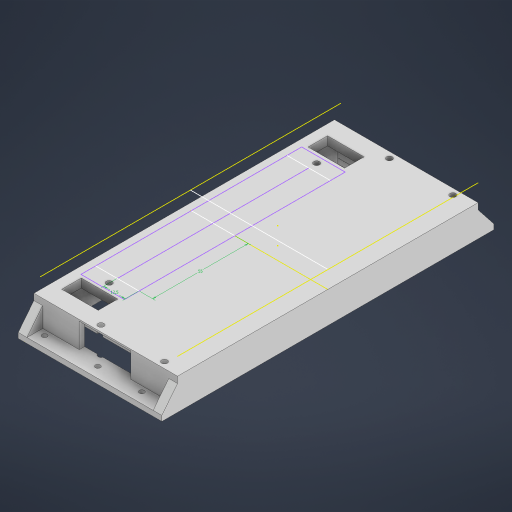
# Autodesk Inventor part: atap
Saved by Autodesk Inventor 2024.3 (Build 283343000, 343)
## iProperties
Created: 2025-06-23
Part Number: atap
Material: Generic
Document SubType Name: Modeling
Designer: Akbar Syihabuddin
Density: 1 g/cm^3
Appearance: Default
Author: Akbar Syihabuddin
Autodesk Inventor part; units mm, degrees
ref_plane "YZ Plane" through (0, 0, 0) normal (1, 0, 0) x (0, 1, 0)
ref_plane "XZ Plane" through (0, 0, 0) normal (0, 1, 0) x (-1, 0, 0)
ref_plane "XY Plane" through (0, 0, 0) normal (0, 0, 1) x (1, 0, 0)
sketch "Sketch1" plane through (0, 0, 0) normal (0, 1, 0) x (-1, 0, 0)
  line L0 (-36.0847, -75.9608) -> (-36.0847, -87.9608)
  line L1 (-36.0847, -87.9608) -> (42.9536, -87.9608)
  line L2 (42.9536, -87.9608) -> (42.9536, -75.9608)
  line L3 (42.9536, -75.9608) -> (-36.0847, -75.9608)
  line L4 (-36.0847, -75.9608) -> (-36.0847, -87.9608)
  circle A0 centre (-18.6075, -81.9608) radius 1.4
  circle A1 centre (-18.6075, -81.9608) radius 1.4
  circle A2 centre (6.6962, -81.9608) radius 1.4
  circle A3 centre (6.6962, -81.9608) radius 1.4
  circle A4 centre (37.2679, -81.9608) radius 1.4
  circle A5 centre (37.2679, -81.9608) radius 1.4
  line L5 (-36.0847, 90.7296) -> (-36.0847, 102.7296)
  line L6 (-36.0847, 102.7296) -> (42.9536, 102.7296)
  line L7 (42.9536, 102.7296) -> (42.9536, 90.7296)
  line L8 (42.9536, 90.7296) -> (-36.0847, 90.7296)
  line L9 (-36.0847, 90.7296) -> (-36.0847, 102.7296)
  circle A6 centre (-18.6075, 96.7296) radius 1.4
  circle A7 centre (-18.6075, 96.7296) radius 1.4
  circle A8 centre (6.6962, 96.7296) radius 1.4
  circle A9 centre (6.6962, 96.7296) radius 1.4
  circle A10 centre (37.2679, 96.7296) radius 1.4
  circle A11 centre (37.2679, 96.7296) radius 1.4
  point P0 (0, 0)
  point P1 (-48.8522, 7.3844)
  constraints: 20 end point, 12 centre point, 6 coincident, 2 parallel, 1 horizontal, 1 perpendicular
extrude "Extrusion1" add sketch "Sketch1" along normal blind 3
sketch "Sketch2" plane through (0, 3, 0) normal (0, 1, 0) x (1, 0, 0)
  line L0 (36.0847, -90.7296) -> (-42.9536, -90.7296) projected
  line L1 (-42.9536, -90.7296) -> (-42.9536, -102.7296) projected
  line L2 (36.0847, -90.7296) -> (-42.9536, -90.7296)
  line L3 (-42.9536, -90.7296) -> (-42.9536, -93.7296)
  line L4 (-42.9536, -93.7296) -> (36.0847, -93.7296)
  line L5 (36.0847, -93.7296) -> (36.0847, -90.7296)
  line L6 (-42.9536, 76.0091) -> (36.0847, 76.0091)
  line L7 (36.0847, 76.0091) -> (36.0847, 79.0091)
  line L8 (36.0847, 79.0091) -> (-42.9536, 79.0091)
  line L9 (-42.9536, 79.0091) -> (-42.9536, 76.0091)
  point P0 (0, 0)
  dimension "d2" = 3
  dimension "d3" = 3
  constraints: 16 end point, 4 parallel, 3 point on line, 2 horizontal, 2 perpendicular
  measures "d2" distance of L3.end L2.end
  measures "d3" distance of L7.end L6.end
extrude "Extrusion2" add sketch "Sketch2" along normal blind 25
sketch "Sketch3" plane through (-42.9536, 3, -76.0091) normal (0, 0, 1) x (1, 0, 0)
  line L0 (0, 0) -> (0, 25) projected
  line L1 (79.0383, 0) -> (79.0383, 25) projected
  line L2 (0, 25) -> (79.0383, 25)
  line L3 (79.0383, 25) -> (79.0383, 20)
  line L4 (79.0383, 20) -> (0, 20)
  line L5 (0, 20) -> (0, 25)
  point P0 (42.9536, -3)
  point P1 (0, 20)
  dimension "d6" = 5
  constraints: 8 end point, 2 parallel, 1 horizontal, 1 perpendicular, 1 point on line
  measures "d6" distance of L2.end L3.end
extrude "Extrusion3" add sketch "Sketch3" along normal blind 168
sketch "Sketch4" plane through (-42.9536, 3, 93.7296) normal (0, 0, 1) x (1, 0, 0)
  line L0 (79.0383, 0) -> (0, 0) projected
  line L1 (22.5307, 0) -> (52.1586, 0)
  line L2 (52.1586, 0) -> (52.1586, 14.1048)
  line L3 (52.1586, 14.1048) -> (22.5307, 14.1048)
  line L4 (22.5307, 14.1048) -> (22.5307, 0)
  point P0 (42.9536, -3)
  constraints: 8 end point, 2 parallel, 1 horizontal, 1 perpendicular, 1 point on line
extrude "Extrusion4" cut sketch "Sketch4" against normal blind 20
sketch "Sketch5" plane through (36.0847, 0, 102.7296) normal (1, 0, 0) x (0, 0, -1)
  line L0 (0, 3) -> (9, 3) projected
  line L1 (0, 3) -> (9, 14.3829)
  line L2 (9, 3) -> (9, 28) projected
  line L3 (0, 0) -> (0, 3) projected
  line L4 (0, 3) -> (9, 3)
  line L5 (9, 14.3829) -> (9, 3)
  point P0 (102.7296, 0)
  constraints: 6 end point, 2 collinear, 1 point on line
extrude "Extrusion5" add sketch "Sketch5" against normal blind 5
sketch "Sketch7" plane through (36.0847, 0, 102.7296) normal (1, 0, 0) x (0, 0, -1)
  line L0 (190.7387, 3) -> (181.7387, 14.3829)
  line L1 (181.7387, 14.3829) -> (190.7387, 3)
  line L2 (181.7387, 3) -> (190.7387, 3)
  line L3 (190.7387, 3) -> (181.7387, 3)
  line L4 (181.7387, 3) -> (181.7387, 14.3829)
  point P0 (102.7296, 0)
  constraints: 10 end point, 1 collinear, 1 horizontal, 1 perpendicular
extrude "Extrusion7" add sketch "Sketch7" against normal blind 5
sketch "Sketch10" plane through (36.0847, 3, -76.0091) normal (0, 0, 1) x (1, 0, 0)
  line L0 (0, -3) -> (0, 0) projected
  line L1 (0, 20) -> (-79.0383, 20) projected
  line L2 (0, -3) -> (-5, -3)
  line L3 (-5, -3) -> (-5, 20)
  line L4 (-5, 20) -> (0, 20)
  line L5 (0, 20) -> (0, -3)
  point P0 (-36.0847, -3)
  point P1 (-74.0383, 20)
  dimension "d22" = 5
  constraints: 8 end point, 2 parallel, 1 horizontal, 1 perpendicular, 1 point on line
  measures "d22" distance of L3.end L4.end
extrude "Extrusion10" add sketch "Sketch10" along normal blind 168
sketch "Sketch11" plane through (0, 28, 0) normal (0, 1, 0) x (1, 0, 0)
  line L0 (-42.9536, 79.0091) -> (-42.9536, -93.7296) projected
  line L1 (-42.9536, -7.3603) -> (36.0847, -7.3603)
  line L2 (36.0847, -93.7296) -> (36.0847, 79.0091) projected
  point P0 (0, 0)
  constraints: 2 end point, 2 midpoint
sketch "Sketch12" plane through (-42.9536, 0, -87.9608) normal (-1, 0, 0) x (0, 0, 1)
  line L0 (0, 0) -> (190.6905, 0) projected
  line L1 (0, 0) -> (0, 3) projected
  line L2 (0, 0) -> (0, 3)
  point P0 (87.9608, 0)
  constraints: 2 end point, 1 vertical
sketch "Sketch13" plane through (-42.9536, 0, 90.7296) normal (-1, 0, 0) x (0, 0, 1)
  line L0 (-178.6905, 0) -> (-178.6905, 3) projected
  line L1 (-178.6905, 0) -> (-178.6905, 3)
  line L2 (-169.7387, 3) -> (-169.7387, 28) projected
  line L3 (-178.6905, 3) -> (-169.7387, 3)
  line L4 (-169.7387, 28) -> (3, 28) projected
  line L5 (-169.7387, 3) -> (-169.7387, 28)
  line L6 (-169.7387, 28) -> (3, 28)
  line L7 (3, 28) -> (3, 3)
  line L8 (12, 0) -> (12, 3) projected
  line L9 (3, 3) -> (12, 3)
  line L10 (12, 3) -> (12, 0)
  line L11 (0, 23) -> (0, 0) projected
  line L12 (12, 0) -> (0, 0)
  line L13 (0, 0) -> (0, 23)
  line L14 (-166.7387, 3) -> (-166.7387, 23) projected
  line L15 (0, 23) -> (-166.7387, 23)
  line L16 (-166.7387, 23) -> (-166.7387, 0)
  line L17 (-166.7387, 0) -> (-178.6905, 0)
  point P0 (-90.7296, 0)
  constraints: 24 end point, 7 perpendicular, 4 collinear, 2 point on line, 1 vertical
extrude "Extrusion11" add sketch "Sketch13" along normal blind 3.5
sketch "Sketch14" plane through (-46.4536, 0, 90.7296) normal (-1, 0, 0) x (0, 0, 1)
  line L0 (-169.7387, 14.3829) -> (-178.7387, 3) projected
  line L1 (12, 3) -> (3, 14.3829) projected
  line L2 (-169.7387, 3) -> (-178.6905, 3) projected
  line L3 (-178.7387, 3) -> (-169.7387, 3)
  line L4 (-169.7387, 3) -> (-169.7387, 14.3829)
  line L5 (-169.7387, 14.3829) -> (-178.7387, 3)
  line L6 (3, 14.3829) -> (3, 3)
  line L7 (3, 3) -> (12, 3)
  line L8 (3, 14.3829) -> (12, 3)
  point P0 (-90.7296, 0)
  constraints: 12 end point, 3 collinear, 2 perpendicular, 2 point on line, 1 parallel
extrude "Extrusion12" add sketch "Sketch14" against normal blind 5
sketch "Sketch15" plane through (31.0847, 0, 90.7296) normal (0, 0, -1) x (-1, 0, 0)
  line L0 (77.5383, 23) -> (77.5383, 0) projected
  line L1 (0, 0) -> (77.5383, 0) projected
  line L2 (77.5383, 23) -> (72.5383, 23)
  line L3 (72.5383, 23) -> (72.5383, 0)
  line L4 (72.5383, 0) -> (77.5383, 0)
  line L5 (77.5383, 0) -> (77.5383, 23)
  point P0 (31.0847, 0)
  dimension "d29" = 5
  constraints: 8 end point, 2 parallel, 1 horizontal, 1 perpendicular, 1 point on line
  measures "d29" distance of L4.end L3.end
extrude "Extrusion13" add sketch "Sketch15" along normal blind 168
sketch "Sketch16" plane through (0, 28, 0) normal (0, 1, 0) x (1, 0, 0)
  line L0 (31.0847, 75.9608) -> (31.0847, -90.7296) projected
  circle A0 centre (31.0847, 72.801) radius 1.65
  circle A1 centre (-37.2679, 72.801) radius 1.65
  circle A2 centre (-6.278, 72.801) radius 1.65
  line L1 (-42.9536, -7.3603) -> (36.0847, -7.3603) projected
  circle A3 centre (31.0847, -87.5216) radius 1.65
  circle A4 centre (-37.2679, -87.5216) radius 1.65
  circle A5 centre (-6.278, -87.5216) radius 1.65
  point P0 (0, 0)
  point P1 (31.0847, -90.6814)
  dimension "d32" = 3.3
  dimension "d33" = 3.3
  constraints: 6 centre point, 4 symmetric about line, 1 point on line, 3 other
  measures "d32" diameter of A0
  measures "d33" diameter of A2
extrude "Extrusion14" cut sketch "Sketch16" against normal blind 168
sketch "Sketch17" plane through (0, 28, 0) normal (0, 1, 0) x (1, 0, 0)
  line L0 (36.0847, 79.0091) -> (-46.4536, 79.0091) projected
  line L1 (31.0847, -93.7296) -> (36.0847, -93.7296) projected
  line L2 (-46.4536, 79.0091) -> (36.0847, 79.0091)
  line L3 (36.0847, 79.0091) -> (36.0847, -93.7296)
  line L4 (36.0847, -93.7296) -> (-46.4536, -93.7296)
  line L5 (-46.4536, -93.7296) -> (-46.4536, 79.0091)
  arc A0 (31.0847, -89.1716) -> (31.0847, -85.8716) centre (31.0847, -87.5216) ccw projected
  circle A1 centre (31.0847, -87.5216) radius 1.65
  circle A2 centre (-6.278, -87.5216) radius 1.65 projected
  circle A3 centre (-6.278, -87.5216) radius 1.65
  circle A4 centre (-37.2679, -87.5216) radius 1.65 projected
  circle A5 centre (-37.2679, -87.5216) radius 1.65
  circle A6 centre (-37.2679, 72.801) radius 1.65 projected
  circle A7 centre (-37.2679, 72.801) radius 1.65
  circle A8 centre (-6.278, 72.801) radius 1.65 projected
  circle A9 centre (-6.278, 72.801) radius 1.65
  arc A10 (31.0847, 71.151) -> (31.0847, 74.451) centre (31.0847, 72.801) ccw projected
  circle A11 centre (31.0847, 72.801) radius 1.65
  point P0 (0, 0)
  point P1 (31.0847, -85.8716)
  constraints: 8 end point, 6 centre point, 6 coincident, 2 parallel, 1 horizontal, 1 perpendicular
extrude "Extrusion15" cut sketch "Sketch17" against normal blind 10
sketch "Sketch18" plane through (-41.4536, 0, 90.7296) normal (1, 0, 0) x (0, 0, -1)
  line L0 (166.7387, 18) -> (0, 18) projected
  line L1 (166.7387, 18) -> (166.7387, 3) projected
  line L2 (0, 18) -> (166.7387, 18)
  line L3 (166.7387, 18) -> (166.7387, 13)
  line L4 (166.7387, 13) -> (0, 13)
  line L5 (0, 13) -> (0, 18)
  point P0 (90.7296, 0)
  dimension "d38" = 5
  constraints: 8 end point, 2 parallel, 1 horizontal, 1 perpendicular, 1 point on line
  measures "d38" distance of L2.end L3.end
extrude "Extrusion16" add sketch "Sketch18" along normal blind 75
sketch "Sketch19" plane through (0, 18, 0) normal (0, 1, 0) x (1, 0, 0)
  line L0 (33.4512, -7.3603) -> (-16.5488, -7.3603)
  line L1 (-16.5488, -7.3603) -> (-16.5488, 69.1397)
  line L2 (-16.5488, 69.1397) -> (33.4512, 69.1397)
  line L3 (33.4512, 69.1397) -> (33.4512, -7.3603)
  line L4 (33.4512, -7.3603) -> (-16.5488, -7.3603)
  line L5 (-16.5488, -7.3603) -> (-16.5488, -83.8603)
  line L6 (-16.5488, -83.8603) -> (33.4512, -83.8603)
  line L7 (33.4512, -83.8603) -> (33.4512, -7.3603)
  line L8 (36.0847, 79.0091) -> (36.0847, -93.7296) projected
  line L9 (36.0847, -7.3603) -> (-18.6839, -7.3603)
  line L10 (-18.6839, -7.3603) -> (-18.6839, -86.5599)
  line L11 (-18.6839, -86.5599) -> (36.0847, -86.5599)
  line L12 (36.0847, -86.5599) -> (36.0847, -7.3603)
  line L13 (-18.6839, 71.8393) -> (36.0847, 71.8393)
  line L14 (-18.6839, -7.3603) -> (-18.6839, 71.8393)
  circle A0 centre (-11.398, -90.2259) radius 1.65
  circle A1 centre (25.0886, -90.2259) radius 1.65
  line L15 (36.0847, -86.5599) -> (36.0847, -93.7296)
  line L16 (36.0847, -93.7296) -> (-18.6839, -93.7296)
  line L17 (-20.4229, -90.7296) -> (9.205, -90.7296) projected
  line L18 (-18.6839, -93.7296) -> (-18.6839, -86.5599)
  line L19 (-18.6839, 71.8393) -> (36.0847, 71.8393)
  circle A2 centre (-11.398, 75.5053) radius 1.65
  circle A3 centre (25.0886, 75.5053) radius 1.65
  line L20 (36.0847, 71.8393) -> (36.0847, 79.0091)
  line L21 (36.0847, 79.0091) -> (-18.6839, 79.0091)
  line L22 (-20.4229, 76.0091) -> (9.205, 76.0091)
  line L23 (-18.6839, 79.0091) -> (-18.6839, 71.8393)
  point P0 (0, 0)
  dimension "d41" = 50
  dimension "d42" = 76.5
  dimension "d43" = 76.5
  dimension "d44" = 3.3
  dimension "d45" = 3.3
  constraints: 44 end point, 7 parallel, 7 symmetric about line, 4 centre point, 4 perpendicular, 3 horizontal, 1 collinear, 1 midpoint, 1 vertical, 2 other
  measures "d41" distance of L1.end L2.end
  measures "d42" distance of L0.end L1.end
  measures "d43" distance of L5.end L4.end
  measures "d44" diameter of A0
  measures "d45" diameter of A1
extrude "Extrusion17" cut sketch "Sketch19" against normal blind 75 contours A2 L22 | L22 A2 | A0 L17 | L17 A0 | A1 | A3
sketch "Sketch20" plane through (0, 18, 0) normal (0, 1, 0) x (1, 0, 0)
  circle A0 centre (-11.398, 75.5053) radius 1.65 projected
  line L0 (-11.398, 75.5053) -> (-37.0391, 75.5053)
  line L1 (-12.9693, 76.0091) -> (-41.4536, 76.0091) projected
  circle A1 centre (-37.0391, 75.5053) radius 1.65
  line L2 (-42.9536, -7.3603) -> (36.0847, -7.3603) projected
  circle A2 centre (-37.0391, -90.2259) radius 1.65
  line L3 (-46.4536, -93.7296) -> (-46.4536, 79.0091) projected
  line L4 (-46.4536, -7.3603) -> (-19.4536, -7.3603)
  line L5 (-19.4536, -7.3603) -> (-40.4536, -7.3603)
  line L6 (-40.4536, -7.3603) -> (-40.4536, 47.6397)
  line L7 (-40.4536, 47.6397) -> (-19.4536, 47.6397)
  line L8 (-19.4536, 47.6397) -> (-19.4536, -7.3603)
  line L9 (-19.4536, -7.3603) -> (-40.4536, -7.3603)
  line L10 (-40.4536, -7.3603) -> (-40.4536, -62.3603)
  line L11 (-40.4536, -62.3603) -> (-19.4536, -62.3603)
  line L12 (-19.4536, -62.3603) -> (-19.4536, -7.3603)
  circle A3 centre (-29.9536, 52.2555) radius 1.65
  line L13 (-29.9536, -62.3603) -> (-29.9536, -66.9763)
  circle A4 centre (-29.9536, -66.9763) radius 1.65
  line L14 (-19.4536, -72.5437) -> (-40.4536, -72.5437)
  line L15 (-40.4536, -72.5437) -> (-40.4536, -83.7487)
  line L16 (-40.4536, -83.7487) -> (-19.4536, -83.7487)
  line L17 (-19.4536, -83.7487) -> (-19.4536, -72.5437)
  line L18 (-19.4536, 57.8231) -> (-40.4536, 57.8231)
  line L19 (-40.4536, 57.8231) -> (-40.4536, 69.0282)
  line L20 (-40.4536, 69.0282) -> (-19.4536, 69.0282)
  line L21 (-19.4536, 69.0282) -> (-19.4536, 57.8231)
  point P0 (0, 0)
  point P1 (-41.4536, -90.7296)
  dimension "d48" = 3.3
  dimension "d49" = 27
  dimension "d50" = 21
  dimension "d51" = 55
  dimension "d52" = 55
  dimension "d53" = 3.3
  dimension "d54" = 4.616
  dimension "d55" = 3.3
  constraints: 38 end point, 7 parallel, 7 symmetric about line, 4 centre point, 3 coincident, 3 horizontal, 3 perpendicular, 2 midpoint, 2 point on line, 1 vertical, 2 other
  measures "d48" diameter of A1
  measures "d49" distance of L4.start L4.end
  measures "d50" distance of L6.end L7.end
  measures "d51" distance of L5.end L6.end
  measures "d52" distance of L10.end L9.end
  measures "d53" diameter of A3
  measures "d54" distance of L13.start L13.end
  measures "d55" diameter of A4
extrude "Extrusion18" cut sketch "Sketch20" against normal blind 75 contours A4 | A3 | L17 L16 L15 L14 | L18 L19 L20 L21
sketch "Sketch21" plane through (0, 18, 0) normal (0, 1, 0) x (1, 0, 0)
  line L0 (-42.9536, -7.3603) -> (36.0847, -7.3603) projected
  line L1 (-29.9536, -7.3603) -> (-17.4536, -7.3603)
  line L2 (-17.4536, -7.3603) -> (-17.4536, -62.3603)
  line L3 (-17.4536, -62.3603) -> (-29.9536, -62.3603)
  line L4 (-29.9536, -62.3603) -> (-29.9536, -7.3603)
  line L5 (-29.9536, -7.3603) -> (-42.4536, -7.3603)
  line L6 (-42.4536, -7.3603) -> (-42.4536, -62.3603)
  line L7 (-42.4536, -62.3603) -> (-29.9536, -62.3603)
  line L8 (-17.4536, -7.3603) -> (-17.4536, 47.6397)
  line L9 (-17.4536, 47.6397) -> (-29.9536, 47.6397)
  line L10 (-29.9536, 47.6397) -> (-29.9536, -7.3603)
  line L11 (-42.4536, -7.3603) -> (-42.4536, 47.6397)
  line L12 (-42.4536, 47.6397) -> (-29.9536, 47.6397)
  line L13 (-17.4536, 47.6397) -> (-42.4536, 47.6397)
  line L14 (-42.4536, 47.6397) -> (-42.4536, 56.0699)
  line L15 (-42.4536, 56.0699) -> (-17.4536, 56.0699)
  line L16 (-17.4536, 56.0699) -> (-17.4536, 47.6397)
  line L17 (-17.4536, -62.3603) -> (-29.9536, -62.3603)
  line L18 (-42.4536, -62.3603) -> (-29.9536, -62.3603)
  line L19 (-17.4536, -62.3603) -> (-42.4536, -62.3603)
  line L20 (-42.4536, -62.3603) -> (-42.4536, -70.7904)
  line L21 (-42.4536, -70.7904) -> (-17.4536, -70.7904)
  line L22 (-17.4536, -70.7904) -> (-17.4536, -62.3603)
  point P0 (0, 0)
  dimension "d58" = 12.5
  dimension "d59" = 55
  constraints: 44 end point, 9 symmetric about line, 4 parallel, 2 horizontal, 2 perpendicular, 1 point on line
  measures "d58" distance of L2.end L3.end
  measures "d59" distance of L1.end L2.end
body "Solid1"
